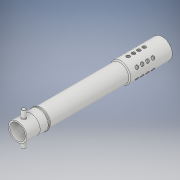
# Autodesk Inventor part: canon
Saved by Autodesk Inventor 2019 (Build 230136000, 136)
## iProperties
Created: 2018-04-25
Part Number: canon
Material: Plastique ABS
Document SubType Name: Modeling
Designer: Theo
Density: 1.06 g/cm^3
Appearance: Lisse - Blanc
Author: Theo
Autodesk Inventor part; units mm, degrees
ref_plane "YZ Plane" through (0, 0, 0) normal (1, 0, 0) x (0, 1, 0)
sketch "Esquisse1" plane through (0, 0, 0) normal (1, 0, 0) x (0, 1, 0)
  line L0 (12, -31.125) -> (12, -134)
  line L1 (12, 0) -> (10.25, 0)
  line L2 (10.25, 0) -> (10.25, -140)
  line L3 (0, 3.9505) -> (0, -129.8897)
  line L4 (10, -5.5573) -> (10, -34.9926) construction
  line L5 (10.25, -140) -> (11.25, -141)
  line L6 (11.25, -141) -> (11.25, -189.75)
  line L7 (11.25, -189.75) -> (11.5, -190)
  line L8 (11.5, -190) -> (13, -190)
  line L9 (13, -190) -> (13.25, -189.75)
  line L10 (13.25, -189.75) -> (13.25, -135.25)
  line L11 (13.25, -135.25) -> (12, -134)
  line L12 (12, -31.125) -> (13, -29.125)
  line L13 (13, -29.125) -> (13, -28.125)
  line L14 (13, -28.125) -> (12.5, -27.625)
  line L15 (12.5, -27.625) -> (12, -17.625)
  line L16 (12, -17.625) -> (12, 0)
  point P0 (0, 0)
  dimension "d0" = 24
  dimension "d1" = 0.25
  dimension "d2" = 20
  dimension "d7" = 1
  dimension "d8" = 1
  dimension "d9" = 0.25
  dimension "d10" = 0.25
  dimension "d11" = 0.25
  dimension "d12" = 0.25
  dimension "d13" = 2
  dimension "d14" = 50
  dimension "d15" = 190
  dimension "d16" = 6
  dimension "d31" = 28.125
  dimension "d32" = 0.5
  dimension "d33" = 0.5
  dimension "d34" = 10
  dimension "d35" = 1
  dimension "d36" = 2
  dimension "d37" = 0.5
  constraints: 34 end point, 7 vertical, 2 horizontal, 1 collinear, 1 horizontal alignment, 1 parallel, 1 perpendicular, 1 point on line
  measures "d0" diameter of L0 L3
  measures "d1" distance between parallel lines of L2 L4
  measures "d2" diameter of L4 L3
  measures "d7" horizontal distance of L2.end L5.end
  measures "d8" horizontal distance of L2.end L5.end
  measures "d9" horizontal distance of L8.end L9.end
  measures "d10" horizontal distance of L8.end L9.end
  measures "d11" horizontal distance of L6.end L7.end
  measures "d12" horizontal distance of L6.end L7.end
  measures "d13" distance between parallel lines of L10 L6
  measures "d14" distance from line of L8 L2.end
  measures "d15" distance between parallel lines of L1 L8
  measures "d16" vertical distance of L0.end L2.end
  measures "d31" distance from line of L13.end L1
  measures "d32" horizontal distance of L13.end L14.end
  measures "d33" horizontal distance of L13.end L14.end
  measures "d34" vertical distance of L14.end L15.end
  measures "d35" distance of L12.end L13.end
  measures "d36" vertical distance of L0.start L12.end
  measures "d37" horizontal distance of L14.end L15.end
revolve "Révolution1" add sketch "Esquisse1" angle 360 about axis through (0, 0, 3.9505) along (0, 0, -1)
ref_plane "Plan de construction1" through (0, -13.25, -162.5) normal (0, 1, 0) x (-1, 0, 0)
sketch "Esquisse2" plane through (0, -13.25, -162.5) normal (0, 1, 0) x (-1, 0, 0)
  line L0 (-11.25, 21.5) -> (11.25, 21.5) projected
  circle A0 centre (0, 17.5) radius 2
  circle A1 centre (0, 10.5) radius 2
  circle A2 centre (0, 3.5) radius 2
  circle A3 centre (0, -3.5) radius 2
  point P0 (0, 162.5)
  dimension "d18" = 4
  dimension "d19" = 7
  dimension "d20" = 7
  dimension "d21" = 4
  dimension "d22" = 7
  constraints: 4 centre point, 3 equal radius
  measures "d18" diameter of A0
  measures "d19" distance of A1.centre A0.centre
  measures "d20" distance of A2.centre A1.centre
  measures "d21" distance from line of L0 A0.centre
  measures "d22" distance of A3.centre A2.centre
extrude "Extrusion1" cut sketch "Esquisse2" along normal up to surface
chamfer "Chanfrein1" distance 0.25 angle 45 16 edges at (2, -11.0708, -151.9978) (-1.5171, -13.1629, -150.6967) (2, -13.0982, -151.9997) (-1.5155, -13.163, -153.3051) (2, -11.0708, -144.9978) (-1.5171, -13.1629, -143.6967) (2, -13.0982, -144.9997) (-1.5155, -13.163, -146.3051) (-1.5171, -13.1629, -157.6967) (2, -13.0982, -158.9997) (-1.5155, -13.163, -160.3051) (2, -11.0708, -158.9978) (-1.5171, -13.1629, -164.6967) (2, -13.0982, -165.9997) (-1.5155, -13.163, -167.3051) (2, -11.0708, -165.9978)
pattern_circular "Réseau circulaire1" count 6 over 360 about axis through (0, 0, -10) along (0, 0, 1) of "Extrusion1", "Chanfrein1"
ref_plane "Plan de construction2" through (0, 12, -8.8125) normal (0, 1, 0) x (-1, 0, 0)
sketch "Esquisse3" plane through (0, 12, -8.8125) normal (0, 1, 0) x (-1, 0, 0)
  line L0 (-12, 8.8125) -> (12, 8.8125) projected
  circle A0 centre (0, 0.8125) radius 2.5
  point P0 (0, 8.8125)
  dimension "d38" = 8
  dimension "d39" = 5
  constraints: 1 centre point
  measures "d38" distance of A0.centre point (0, 8.812)
  measures "d39" diameter of A0
extrude "Extrusion2" add sketch "Esquisse3" along normal blind 10 and the other way blind 1
chamfer "Chanfrein2" distance 0.5 angle 45 4 edges at (2.5, 11.7367, -7.9997) (-1.9013, 11.8484, -6.3767) (-1.9003, 11.8486, -9.6245) (2.5, 22, -8)
pattern_circular "Réseau circulaire2" count 2 over 360 about axis through (0, 0, -10) along (0, 0, 1) of "Extrusion2", "Chanfrein2"
equation "\"d10\" = d9"
equation "\"d11\" = d9"
equation "\"d12\" = d9"
equation "\"d33\" = d32"
equation "\"d20\" = d19"
equation "\"d22\" = d19"
